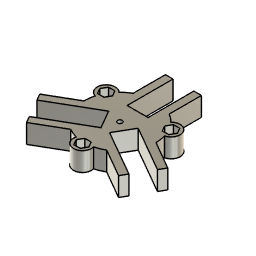
Gripper Assembly v1 (Autodesk Fusion 360 archive; units mm, degrees)
design "Front base"
Autodesk Fusion 360 part; units mm, degrees
sketch "Sketch1" plane through (0, 0, 0) normal (0, 0, 1) x (1, 0, 0)
  line L0 (5, 35) -> (45, 35)
  line L1 (45, 35) -> (45, -135.4224)
  line L2 (5, -135.4224) -> (5, 35)
  spline S0 degree 5 poles (45, -135.4224) (45.4605, -135.6915) (46.3795, -136.2324) (47.752, -137.0519) (49.5701, -138.1606) (51.8226, -139.5739) (54.0546, -141.0154) (56.2658, -142.4857) (58.4561, -143.9858) (60.6259, -145.5165) (62.7755, -147.0783) (64.9051, -148.6715) (67.0143, -150.296) (69.1022, -151.9513) (71.1668, -153.6357) (73.2054, -155.3473) (75.2154, -157.0838) (77.194, -158.8431) (79.1392, -160.6231) (81.0502, -162.4223) (82.9268, -164.2396) (84.4008, -165.7074) (85.491, -166.8158) (86.2111, -167.5582) (86.5694, -167.9302) knots 0 0 0 0 0 0 0.05 0.1 0.15 0.2 0.25 0.3 0.35 0.4 0.45 0.5 0.55 0.6 0.65 0.7 0.75 0.8 0.85 0.9 0.95 1 1 1 1 1 1
  circle A0 centre (121, -201) radius 17.4626
  line L3 (287.62, -385.23) -> (140, -300)
  line L4 (119.9736, -334.6861) -> (267.6136, -419.8616)
  line L5 (267.6136, -419.8616) -> (287.62, -385.23)
  line L6 (119.9736, -334.6861) -> (27.9247, -281.5818)
  line L7 (27.9247, -281.5818) -> (-27.2814, -377.2739)
  line L8 (-27.2814, -377.2739) -> (212.617, -515.1318)
  line L9 (212.617, -515.1318) -> (192.6182, -549.7743)
  line L10 (192.6182, -549.7743) -> (45.092, -464.6088)
  line L11 (5, -135.4224) -> (5, -206.756)
  line L12 (-50, -206.756) -> (5, -206.756)
  spline S1 degree 5 poles (132.5048, -247.3327) (132.6447, -247.7867) (132.9219, -248.702) (133.3302, -250.0971) (133.8594, -252.0018) (134.4952, -254.4571) (135.1045, -256.9868) (135.6863, -259.5888) (136.2394, -262.2585) (136.7623, -264.9875) (137.2534, -267.7647) (137.711, -270.5775) (138.133, -273.4114) (138.5175, -276.2513) (138.8621, -279.082) (139.1649, -281.8886) (139.4238, -284.6572) (139.6373, -287.3762) (139.8044, -290.0362) (139.9248, -292.6319) (139.999, -295.1607) (140.0219, -297.1299) (140.0188, -298.5766) (140.0078, -299.5278) (140, -300) knots 0 0 0 0 0 0 0.05 0.1 0.15 0.2 0.25 0.3 0.35 0.4 0.45 0.5 0.55 0.6 0.65 0.7 0.75 0.8 0.85 0.9 0.95 1 1 1 1 1 1
  spline S2 degree 5 poles (45.092, -464.6088) (44.6241, -464.8703) (43.6871, -465.3905) (42.2779, -466.1627) (40.3917, -467.1758) (38.0214, -468.414) (35.6384, -469.6236) (33.2422, -470.8036) (30.8324, -471.9529) (28.4086, -473.0708) (25.9704, -474.1561) (23.5176, -475.208) (21.0501, -476.2257) (18.568, -477.2083) (16.0719, -478.1551) (13.5623, -479.0659) (11.0402, -479.9402) (8.5062, -480.7781) (5.9613, -481.5796) (3.4059, -482.3453) (0.8406, -483.0761) (-1.2193, -483.6331) (-2.7685, -484.0357) (-3.8032, -484.2974) (-4.321, -484.4265) knots 0 0 0 0 0 0 0.05 0.1 0.15 0.2 0.25 0.3 0.35 0.4 0.45 0.5 0.55 0.6 0.65 0.7 0.75 0.8 0.85 0.9 0.95 1 1 1 1 1 1
  arc A1 (132.5048, -247.3327) -> (86.5694, -167.9302) centre (121, -201) ccw
  arc A2 (-50, -545.0131) -> (-4.321, -484.4265) centre (-50, -497.5) ccw
  arc A3 (-50, -515) -> (-50, -480) centre (-50, -497.5) ccw
  line L13 (-145, 35) -> (-145, -135.4224)
  line L14 (-105, 35) -> (-145, 35)
  line L15 (-105, -135.4224) -> (-105, 35)
  line L16 (-105, -135.4224) -> (-105, -206.756)
  line L17 (-50, -206.756) -> (-105, -206.756)
  line L18 (-219.9736, -334.6861) -> (-367.6136, -419.8616)
  line L19 (-219.9736, -334.6861) -> (-127.9247, -281.5818)
  arc A4 (-186.5694, -167.9302) -> (-232.5048, -247.3327) centre (-221, -201) ccw
  spline S3 degree 5 poles (-145, -135.4224) (-145.4605, -135.6915) (-146.3795, -136.2324) (-147.752, -137.0519) (-149.5701, -138.1606) (-151.8226, -139.5739) (-154.0546, -141.0154) (-156.2658, -142.4857) (-158.4561, -143.9858) (-160.6259, -145.5165) (-162.7755, -147.0783) (-164.9051, -148.6715) (-167.0143, -150.296) (-169.1022, -151.9513) (-171.1668, -153.6357) (-173.2054, -155.3473) (-175.2154, -157.0838) (-177.194, -158.8431) (-179.1392, -160.6231) (-181.0502, -162.4223) (-182.9268, -164.2396) (-184.4008, -165.7074) (-185.491, -166.8158) (-186.2111, -167.5582) (-186.5694, -167.9302) knots 0 0 0 0 0 0 0.05 0.1 0.15 0.2 0.25 0.3 0.35 0.4 0.45 0.5 0.55 0.6 0.65 0.7 0.75 0.8 0.85 0.9 0.95 1 1 1 1 1 1
  line L20 (40.1828, -132.6073) -> (49.8172, -138.2376)
  line L21 (82.7521, -163.9673) -> (90.3868, -171.893)
  line L22 (-140.1828, -132.6073) -> (-149.8172, -138.2376)
  line L23 (-182.7521, -163.9673) -> (-190.3868, -171.893)
  spline S4 degree 5 poles (-232.5048, -247.3327) (-232.6447, -247.7867) (-232.9219, -248.702) (-233.3302, -250.0971) (-233.8594, -252.0018) (-234.4952, -254.4571) (-235.1045, -256.9868) (-235.6863, -259.5888) (-236.2394, -262.2585) (-236.7623, -264.9875) (-237.2534, -267.7647) (-237.711, -270.5775) (-238.133, -273.4114) (-238.5175, -276.2513) (-238.8621, -279.082) (-239.1649, -281.8886) (-239.4238, -284.6572) (-239.6373, -287.3762) (-239.8044, -290.0362) (-239.9248, -292.6319) (-239.999, -295.1607) (-240.0219, -297.1299) (-240.0188, -298.5766) (-240.0078, -299.5278) (-240, -300) knots 0 0 0 0 0 0 0.05 0.1 0.15 0.2 0.25 0.3 0.35 0.4 0.45 0.5 0.55 0.6 0.65 0.7 0.75 0.8 0.85 0.9 0.95 1 1 1 1 1 1
  line L24 (130.9887, -242.4116) -> (134.0209, -252.2537)
  line L25 (140.0843, -294.8664) -> (139.9157, -305.1336)
  line L26 (-230.9887, -242.4116) -> (-234.0209, -252.2537)
  line L27 (-240.0843, -294.8664) -> (-239.9157, -305.1336)
  line L28 (-387.62, -385.23) -> (-240, -300)
  line L29 (-367.6136, -419.8616) -> (-387.62, -385.23)
  line L30 (-127.9247, -281.5818) -> (-72.7186, -377.2739)
  line L31 (-72.7186, -377.2739) -> (-312.617, -515.1318)
  line L32 (-312.617, -515.1318) -> (-292.6182, -549.7743)
  line L33 (-292.6182, -549.7743) -> (-145.092, -464.6088)
  spline S5 degree 5 poles (-145.092, -464.6088) (-144.6241, -464.8703) (-143.6871, -465.3905) (-142.2779, -466.1627) (-140.3917, -467.1758) (-138.0214, -468.414) (-135.6384, -469.6236) (-133.2422, -470.8036) (-130.8324, -471.9529) (-128.4086, -473.0708) (-125.9704, -474.1561) (-123.5176, -475.208) (-121.0501, -476.2257) (-118.568, -477.2083) (-116.0719, -478.1551) (-113.5623, -479.0659) (-111.0402, -479.9402) (-108.5062, -480.7781) (-105.9613, -481.5796) (-103.4059, -482.3453) (-100.8406, -483.0761) (-98.7807, -483.6331) (-97.2315, -484.0357) (-96.1968, -484.2974) (-95.679, -484.4265) knots 0 0 0 0 0 0 0.05 0.1 0.15 0.2 0.25 0.3 0.35 0.4 0.45 0.5 0.55 0.6 0.65 0.7 0.75 0.8 0.85 0.9 0.95 1 1 1 1 1 1
  line L34 (49.9585, -461.8889) -> (40.2255, -467.3286)
  line L35 (1.0783, -483.0799) -> (-9.7202, -485.7731)
  line L36 (-149.9585, -461.8889) -> (-140.2255, -467.3286)
  line L37 (-101.0783, -483.0799) -> (-90.2798, -485.7731)
  arc A5 (-95.679, -484.4265) -> (-50, -545.0131) centre (-50, -497.5) ccw
  arc A6 (-50, -480) -> (-50, -515) centre (-50, -497.5) ccw
  circle A7 centre (-221, -201) radius 17.4626
  circle A8 centre (-50, -300) radius 12.5
  line L38 (137.782, -230.2475) -> (154.5192, -201.2524)
  line L39 (154.5192, -201.2524) -> (137.7773, -172.2599)
  line L40 (137.7773, -172.2599) -> (104.2982, -172.2626)
  line L41 (104.2982, -172.2626) -> (87.561, -201.2578)
  line L42 (87.561, -201.2578) -> (104.3029, -230.2502)
  line L43 (104.3029, -230.2502) -> (137.782, -230.2475)
  line L44 (-204.2982, -172.2626) -> (-187.561, -201.2578)
  line L45 (-187.561, -201.2578) -> (-204.3029, -230.2502)
  line L46 (-204.3029, -230.2502) -> (-237.782, -230.2475)
  line L47 (-237.782, -230.2475) -> (-254.5192, -201.2524)
  line L48 (-254.5192, -201.2524) -> (-237.7773, -172.2599)
  line L49 (-237.7773, -172.2599) -> (-204.2982, -172.2626)
  line L50 (-33.2504, -526.5073) -> (-16.5012, -497.5063)
  line L51 (-16.5012, -497.5063) -> (-33.2422, -468.5005)
  line L52 (-33.2422, -468.5005) -> (-66.7325, -468.4957)
  line L53 (-66.7325, -468.4957) -> (-83.4817, -497.4968)
  line L54 (-83.4817, -497.4968) -> (-66.7407, -526.5025)
  line L55 (-66.7407, -526.5025) -> (-33.2504, -526.5073)
  point P0 (56.3101, -142.5266)
  point P1 (67.0964, -150.3721)
  point P2 (77.3051, -158.9561)
  point P3 (135.5465, -258.9948)
  point P4 (138.1258, -273.4283)
  point P5 (139.6709, -288.0188)
  point P6 (33.22, -470.805)
  point P7 (21.0316, -476.2229)
  point P8 (8.4925, -480.7725)
  point P9 (-156.3101, -142.5266)
  point P10 (-167.0964, -150.3721)
  point P11 (-177.3051, -158.9561)
  point P12 (-235.5465, -258.9948)
  point P13 (-238.1258, -273.4283)
  point P14 (-239.6709, -288.0188)
  point P15 (-133.22, -470.805)
  point P16 (-121.0316, -476.2229)
  point P17 (-108.4925, -480.7725)
  point P18 (121.0401, -201.2551)
  point P19 (-49.9914, -497.5015)
  dimension "d4" = 25
  constraint horizontal L0
  constraint vertical L1
  constraint vertical L2
  constraint concentric A0 A1
  constraint perpendicular L6 L7
  constraint perpendicular L9 L10
  constraint concentric A2 A3
  constraint perpendicular L11 L12
  constraint midpoint L1.end L20
  constraint midpoint S0.end L21
  constraint midpoint S1.start L24
  constraint midpoint L3.end L25
  constraint midpoint L10.end L34
  constraint midpoint S2.end L35
  measures "d4" diameter of A8
extrude "Extrude2" add sketch "Sketch1" along normal blind 100 contours L0 L1 L2 S0 L3 L4 L5 L6 L7 L8 L9 L10 L11 L12 S1 S2 A1 A2 L13 L14 L15 L16 L17 L18 L19 A4 S3 S4 L28 L29 L30 L31 L32 L33 S5 A5
scale "Scale2" factor 0.2 about (86.5694, -167.9302, 100) bodies 1

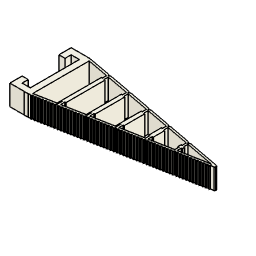
design "CORRUGATED ADAPTIVE FINGER"
Autodesk Fusion 360 part; units mm, degrees
other "Base Mesh Feature1"
sketch "Sketch1" plane through (0, 0, 0) normal (0, 0, 1) x (1, 0, 0)
  line L0 (-20, 150) -> (0, 150)
  line L1 (-0.0012, -150.0012) -> (-19.994, -150.0012)
  line L2 (-90, 150) -> (-20, 150)
  line L3 (-19.994, 120) -> (-60, 120)
  line L4 (-90, 120) -> (-90, 150)
  line L5 (-90, 120) -> (-90, 90)
  line L6 (-90, 90) -> (-60, 90)
  line L7 (-60, 90) -> (-60, 120)
  line L8 (-90, -90) -> (-60, -90)
  line L9 (-60, -90) -> (-60, -120)
  line L10 (-90, -120) -> (-90, -90)
  line L11 (-19.994, -120) -> (-60, -120)
  line L12 (-90, -120) -> (-90, -150)
  line L13 (-90, -150) -> (-19.994, -150)
  line L14 (162.7867, 120.1326) -> (764.7489, 6.3258)
  line L15 (768.431, -1.1614) -> (768.4129, 1.9305)
  line L16 (11.0558, -148.3913) -> (14.7932, -152.3145)
  line L17 (14.7932, -152.3145) -> (16.416, -147.4373)
  line L18 (28.359, -149.753) -> (29.9819, -144.8758)
  line L19 (24.6216, -145.8298) -> (28.359, -149.753)
  line L20 (41.9249, -147.1915) -> (43.5477, -142.3143)
  line L21 (38.1874, -143.2682) -> (41.9249, -147.1915)
  line L22 (55.4907, -144.6299) -> (57.1135, -139.7527)
  line L23 (51.7533, -140.7067) -> (55.4907, -144.6299)
  line L24 (69.0565, -142.0684) -> (70.6794, -137.1912)
  line L25 (65.3191, -138.1452) -> (69.0565, -142.0684)
  line L26 (82.6224, -139.5069) -> (84.2452, -134.6297)
  line L27 (78.885, -135.5837) -> (82.6224, -139.5069)
  line L28 (96.1882, -136.9454) -> (97.811, -132.0682)
  line L29 (92.4508, -133.0221) -> (96.1882, -136.9454)
  line L30 (109.754, -134.3838) -> (111.5052, -129.1209)
  line L31 (106.0166, -130.4606) -> (109.754, -134.3838)
  line L32 (123.3199, -131.8223) -> (124.9427, -126.9451)
  line L33 (119.2419, -127.5416) -> (123.3199, -131.8223)
  line L34 (136.8857, -129.2608) -> (138.5086, -124.3836)
  line L35 (133.1483, -125.3376) -> (136.8857, -129.2608)
  line L36 (150.4516, -126.6993) -> (152.0744, -121.8221)
  line L37 (146.7141, -122.776) -> (150.4516, -126.6993)
  line L38 (164.0174, -124.1377) -> (165.6402, -119.2605)
  line L39 (160.28, -120.2145) -> (164.0174, -124.1377)
  line L40 (177.5832, -121.5762) -> (179.2061, -116.699)
  line L41 (173.8458, -117.653) -> (177.5832, -121.5762)
  line L42 (191.1491, -119.0147) -> (192.7719, -114.1375)
  line L43 (187.4117, -115.0915) -> (191.1491, -119.0147)
  line L44 (204.7149, -116.4532) -> (206.3377, -111.576)
  line L45 (200.9775, -112.5299) -> (204.7149, -116.4532)
  line L46 (218.2807, -113.8916) -> (219.9036, -109.0144)
  line L47 (214.5433, -109.9684) -> (218.2807, -113.8916)
  line L48 (231.8466, -111.3301) -> (233.5929, -106.0817)
  line L49 (228.1092, -107.4069) -> (231.8466, -111.3301)
  line L50 (245.4124, -108.7686) -> (247.0353, -103.8914)
  line L51 (241.4011, -104.5578) -> (245.4124, -108.7686)
  line L52 (258.9783, -106.2071) -> (260.6011, -101.3298)
  line L53 (255.2408, -102.2838) -> (258.9783, -106.2071)
  line L54 (272.5441, -103.6455) -> (274.1669, -98.7683)
  line L55 (268.8067, -99.7223) -> (272.5441, -103.6455)
  line L56 (286.1099, -101.084) -> (287.7328, -96.2068)
  line L57 (282.3725, -97.1608) -> (286.1099, -101.084)
  line L58 (299.6758, -98.5225) -> (301.2986, -93.6453)
  line L59 (295.9384, -94.5993) -> (299.6758, -98.5225)
  line L60 (313.2416, -95.9609) -> (314.8644, -91.0837)
  line L61 (309.5042, -92.0377) -> (313.2416, -95.9609)
  line L62 (326.8074, -93.3994) -> (328.4303, -88.5222)
  line L63 (323.07, -89.4762) -> (326.8074, -93.3994)
  line L64 (340.3733, -90.8379) -> (341.9961, -85.9607)
  line L65 (336.6359, -86.9147) -> (340.3733, -90.8379)
  line L66 (353.9391, -88.2764) -> (355.6866, -83.0245)
  line L67 (350.2017, -84.3531) -> (353.9391, -88.2764)
  line L68 (367.505, -85.7148) -> (369.1278, -80.8376)
  line L69 (363.5002, -81.5109) -> (367.505, -85.7148)
  line L70 (381.0708, -83.1533) -> (382.6936, -78.2761)
  line L71 (377.3334, -79.2301) -> (381.0708, -83.1533)
  line L72 (394.6366, -80.5918) -> (396.2595, -75.7146)
  line L73 (390.8992, -76.6686) -> (394.6366, -80.5918)
  line L74 (408.2025, -78.0303) -> (409.8253, -73.1531)
  line L75 (404.4651, -74.107) -> (408.2025, -78.0303)
  line L76 (421.7683, -75.4687) -> (423.3911, -70.5915)
  line L77 (418.0309, -71.5455) -> (421.7683, -75.4687)
  line L78 (435.3341, -72.9072) -> (436.957, -68.03)
  line L79 (431.5967, -68.984) -> (435.3341, -72.9072)
  line L80 (448.9, -70.3457) -> (450.5228, -65.4685)
  line L81 (445.1626, -66.4225) -> (448.9, -70.3457)
  line L82 (462.4658, -67.7842) -> (464.0887, -62.907)
  line L83 (458.7284, -63.8609) -> (462.4658, -67.7842)
  line L84 (476.0317, -65.2226) -> (477.8401, -59.7876)
  line L85 (472.2942, -61.2994) -> (476.0317, -65.2226)
  line L86 (489.5975, -62.6611) -> (491.2203, -57.7839)
  line L87 (485.4849, -58.3441) -> (489.5975, -62.6611)
  line L88 (503.1633, -60.0996) -> (504.7862, -55.2224)
  line L89 (499.4259, -56.1764) -> (503.1633, -60.0996)
  line L90 (516.7292, -57.5381) -> (518.352, -52.6608)
  line L91 (512.9918, -53.6148) -> (516.7292, -57.5381)
  line L92 (530.295, -54.9765) -> (531.9178, -50.0993)
  line L93 (526.5576, -51.0533) -> (530.295, -54.9765)
  line L94 (543.8608, -52.415) -> (545.4837, -47.5378)
  line L95 (540.1234, -48.4918) -> (543.8608, -52.415)
  line L96 (557.4267, -49.8535) -> (559.0495, -44.9763)
  line L97 (553.6893, -45.9303) -> (557.4267, -49.8535)
  line L98 (570.9925, -47.292) -> (572.6154, -42.4147)
  line L99 (567.2551, -43.3687) -> (570.9925, -47.292)
  line L100 (584.5584, -44.7304) -> (586.1812, -39.8532)
  line L101 (580.8209, -40.8072) -> (584.5584, -44.7304)
  line L102 (598.1242, -42.1689) -> (599.9326, -36.7339)
  line L103 (594.3868, -38.2457) -> (598.1242, -42.1689)
  line L104 (611.69, -39.6074) -> (613.3129, -34.7302)
  line L105 (607.5775, -35.2904) -> (611.69, -39.6074)
  line L106 (625.2559, -37.0458) -> (626.8787, -32.1686)
  line L107 (621.5185, -33.1226) -> (625.2559, -37.0458)
  line L108 (638.8217, -34.4843) -> (640.4445, -29.6071)
  line L109 (635.0843, -30.5611) -> (638.8217, -34.4843)
  line L110 (652.3875, -31.9228) -> (654.0104, -27.0456)
  line L111 (648.6501, -27.9996) -> (652.3875, -31.9228)
  line L112 (665.9534, -29.3613) -> (667.5762, -24.4841)
  line L113 (662.216, -25.438) -> (665.9534, -29.3613)
  line L114 (679.5192, -26.7997) -> (681.1421, -21.9225)
  line L115 (675.7818, -22.8765) -> (679.5192, -26.7997)
  line L116 (693.0851, -24.2382) -> (694.7079, -19.361)
  line L117 (689.3476, -20.315) -> (693.0851, -24.2382)
  line L118 (706.6509, -21.6767) -> (708.2737, -16.7995)
  line L119 (702.9135, -17.7535) -> (706.6509, -21.6767)
  line L120 (720.2167, -19.1152) -> (721.8396, -14.238)
  line L121 (716.4793, -15.1919) -> (720.2167, -19.1152)
  line L122 (733.7826, -16.5536) -> (735.4054, -11.6764)
  line L123 (730.0452, -12.6304) -> (733.7826, -16.5536)
  line L124 (747.3484, -13.9921) -> (749.1569, -8.5571)
  line L125 (743.611, -10.0689) -> (747.3484, -13.9921)
  line L126 (749.1569, -8.5571) -> (764.766, -5.6097)
  line L127 (736.1687, -11.0095) -> (742.7014, -9.776)
  line L128 (722.6029, -13.571) -> (729.1356, -12.3375)
  line L129 (709.037, -16.1326) -> (715.5697, -14.8991)
  line L130 (695.4712, -18.6941) -> (702.0039, -17.4606)
  line L131 (681.9054, -21.2556) -> (688.4381, -20.0221)
  line L132 (668.3395, -23.8171) -> (674.8722, -22.5836)
  line L133 (654.7737, -26.3787) -> (661.3064, -25.1452)
  line L134 (641.2079, -28.9402) -> (647.7405, -27.7067)
  line L135 (627.642, -31.5017) -> (634.1747, -30.2682)
  line L136 (614.0762, -34.0633) -> (620.6089, -32.8297)
  line L137 (586.9445, -39.1863) -> (593.4772, -37.9528)
  line L138 (573.3787, -41.7478) -> (579.9114, -40.5143)
  line L139 (559.8128, -44.3094) -> (566.3455, -43.0758)
  line L140 (546.247, -46.8709) -> (552.7797, -45.6374)
  line L141 (532.6812, -49.4324) -> (539.2138, -48.1989)
  line L142 (519.1153, -51.9939) -> (525.648, -50.7604)
  line L143 (505.5495, -54.5555) -> (512.0822, -53.3219)
  line L144 (491.9836, -57.117) -> (498.5163, -55.8835)
  line L145 (464.852, -62.24) -> (471.3847, -61.0065)
  line L146 (451.2861, -64.8016) -> (457.8188, -63.5681)
  line L147 (437.7203, -67.3631) -> (444.253, -66.1296)
  line L148 (424.1545, -69.9246) -> (430.6871, -68.6911)
  line L149 (410.5886, -72.4861) -> (417.1213, -71.2526)
  line L150 (397.0228, -75.0477) -> (403.5555, -73.8142)
  line L151 (383.4569, -77.6092) -> (389.9896, -76.3757)
  line L152 (9.9848, -148.1289) -> (10.1462, -148.0984)
  line L153 (17.1793, -146.7704) -> (23.712, -145.5369)
  line L154 (30.7452, -144.2089) -> (37.2778, -142.9754)
  line L155 (44.311, -141.6474) -> (50.8437, -140.4138)
  line L156 (57.8768, -139.0858) -> (64.4095, -137.8523)
  line L157 (71.4427, -136.5243) -> (77.9754, -135.2908)
  line L158 (85.0085, -133.9628) -> (91.5412, -132.7293)
  line L159 (98.5744, -131.4012) -> (105.107, -130.1677)
  line L160 (125.706, -126.2782) -> (132.2387, -125.0447)
  line L161 (139.2719, -123.7167) -> (145.8045, -122.4832)
  line L162 (152.8377, -121.1551) -> (159.3704, -119.9216)
  line L163 (166.4035, -118.5936) -> (172.9362, -117.3601)
  line L164 (179.9694, -116.0321) -> (186.5021, -114.7986)
  line L165 (193.5352, -113.4706) -> (200.0679, -112.2371)
  line L166 (207.1011, -110.909) -> (213.6337, -109.6755)
  line L167 (369.8911, -80.1707) -> (376.4238, -78.9372)
  line L168 (342.7594, -85.2938) -> (349.2921, -84.0603)
  line L169 (329.1936, -87.8553) -> (335.7263, -86.6218)
  line L170 (315.6278, -90.4168) -> (322.1604, -89.1833)
  line L171 (302.0619, -92.9784) -> (308.5946, -91.7448)
  line L172 (288.4961, -95.5399) -> (295.0288, -94.3064)
  line L173 (274.9302, -98.1014) -> (281.4629, -96.8679)
  line L174 (261.3644, -100.6629) -> (267.8971, -99.4294)
  line L175 (247.7986, -103.2245) -> (254.3313, -101.9909)
  line L176 (220.6669, -108.3475) -> (227.1996, -107.114)
  line L177 (-19.994, -150.0012) -> (-19.994, -150)
  line L178 (-19.994, -120) -> (-19.994, 120)
  line L179 (9.9848, -148.1289) -> (-0.0012, -150.0012)
  line L180 (162.7867, 120.1326) -> (0, 150)
  line L181 (10, -137.9994) -> (745.7473, -0.0019)
  line L182 (745.7473, -0.0019) -> (10.003, 137.9556)
  line L183 (10.003, 137.9556) -> (10, -137.9994)
  line L184 (607.5775, -35.2904) -> (602, -32)
  line L185 (602, -32) -> (599.9326, -36.7339)
  line L186 (485.4849, -58.3441) -> (480.1362, -55.5815)
  line L187 (480.1362, -55.5815) -> (477.8401, -59.7876)
  line L188 (363.2553, -81.323) -> (359, -79)
  line L189 (359, -79) -> (355.8723, -82.694)
  line L190 (241.1723, -104.3789) -> (237, -102)
  line L191 (237, -102) -> (233.7832, -105.7459)
  line L192 (119.1693, -127.4727) -> (115.3849, -124.2227)
  line L193 (115.3849, -124.2227) -> (111.6766, -128.8078)
  arc A0 (743.611, -10.0689) -> (742.7014, -9.776) centre (742.8869, -10.7586) ccw
  arc A1 (736.1687, -11.0095) -> (735.4054, -11.6764) centre (736.3543, -11.9922) ccw
  arc A2 (730.0452, -12.6304) -> (729.1356, -12.3375) centre (729.3211, -13.3202) ccw
  arc A3 (722.6029, -13.571) -> (721.8396, -14.238) centre (722.7884, -14.5537) ccw
  arc A4 (716.4793, -15.1919) -> (715.5697, -14.8991) centre (715.7553, -15.8817) ccw
  arc A5 (709.037, -16.1326) -> (708.2737, -16.7995) centre (709.2226, -17.1152) ccw
  arc A6 (702.9135, -17.7535) -> (702.0039, -17.4606) centre (702.1894, -18.4432) ccw
  arc A7 (695.4712, -18.6941) -> (694.7079, -19.361) centre (695.6567, -19.6767) ccw
  arc A8 (689.3476, -20.315) -> (688.4381, -20.0221) centre (688.6236, -21.0047) ccw
  arc A9 (681.9054, -21.2556) -> (681.1421, -21.9225) centre (682.0909, -22.2383) ccw
  arc A10 (675.7818, -22.8765) -> (674.8722, -22.5836) centre (675.0578, -23.5663) ccw
  arc A11 (668.3395, -23.8171) -> (667.5762, -24.4841) centre (668.5251, -24.7998) ccw
  arc A12 (662.216, -25.438) -> (661.3064, -25.1452) centre (661.4919, -26.1278) ccw
  arc A13 (654.7737, -26.3787) -> (654.0104, -27.0456) centre (654.9592, -27.3613) ccw
  arc A14 (648.6501, -27.9996) -> (647.7405, -27.7067) centre (647.9261, -28.6893) ccw
  arc A15 (641.2079, -28.9402) -> (640.4445, -29.6071) centre (641.3934, -29.9228) ccw
  arc A16 (635.0843, -30.5611) -> (634.1747, -30.2682) centre (634.3602, -31.2508) ccw
  arc A17 (627.642, -31.5017) -> (626.8787, -32.1686) centre (627.8276, -32.4844) ccw
  arc A18 (621.5185, -33.1226) -> (620.6089, -32.8297) centre (620.7944, -33.8124) ccw
  arc A19 (614.0762, -34.0633) -> (613.3129, -34.7302) centre (614.2617, -35.0459) ccw
  arc A20 (594.3868, -38.2457) -> (593.4772, -37.9528) centre (593.6627, -38.9354) ccw
  arc A21 (586.9445, -39.1863) -> (586.1812, -39.8532) centre (587.13, -40.1689) ccw
  arc A22 (580.8209, -40.8072) -> (579.9114, -40.5143) centre (580.0969, -41.497) ccw
  arc A23 (573.3787, -41.7478) -> (572.6154, -42.4147) centre (573.5642, -42.7305) ccw
  arc A24 (567.2551, -43.3687) -> (566.3455, -43.0758) centre (566.5311, -44.0585) ccw
  arc A25 (559.8128, -44.3094) -> (559.0495, -44.9763) centre (559.9984, -45.292) ccw
  arc A26 (553.6893, -45.9303) -> (552.7797, -45.6374) centre (552.9652, -46.62) ccw
  arc A27 (546.247, -46.8709) -> (545.4837, -47.5378) centre (546.4325, -47.8535) ccw
  arc A28 (540.1234, -48.4918) -> (539.2138, -48.1989) centre (539.3994, -49.1815) ccw
  arc A29 (532.6812, -49.4324) -> (531.9178, -50.0993) centre (532.8667, -50.415) ccw
  arc A30 (526.5576, -51.0533) -> (525.648, -50.7604) centre (525.8335, -51.7431) ccw
  arc A31 (519.1153, -51.9939) -> (518.352, -52.6608) centre (519.3009, -52.9766) ccw
  arc A32 (512.9918, -53.6148) -> (512.0822, -53.3219) centre (512.2677, -54.3046) ccw
  arc A33 (505.5495, -54.5555) -> (504.7862, -55.2224) centre (505.735, -55.5381) ccw
  arc A34 (499.4259, -56.1764) -> (498.5163, -55.8835) centre (498.7019, -56.8661) ccw
  arc A35 (491.9836, -57.117) -> (491.2203, -57.7839) centre (492.1692, -58.0996) ccw
  arc A36 (472.2942, -61.2994) -> (471.3847, -61.0065) centre (471.5702, -61.9892) ccw
  arc A37 (464.852, -62.24) -> (464.0887, -62.907) centre (465.0375, -63.2227) ccw
  arc A38 (458.7284, -63.8609) -> (457.8188, -63.5681) centre (458.0044, -64.5507) ccw
  arc A39 (451.2861, -64.8016) -> (450.5228, -65.4685) centre (451.4717, -65.7842) ccw
  arc A40 (445.1626, -66.4225) -> (444.253, -66.1296) centre (444.4385, -67.1122) ccw
  arc A41 (437.7203, -67.3631) -> (436.957, -68.03) centre (437.9058, -68.3457) ccw
  arc A42 (431.5967, -68.984) -> (430.6871, -68.6911) centre (430.8727, -69.6737) ccw
  arc A43 (424.1545, -69.9246) -> (423.3911, -70.5915) centre (424.34, -70.9073) ccw
  arc A44 (418.0309, -71.5455) -> (417.1213, -71.2526) centre (417.3068, -72.2353) ccw
  arc A45 (410.5886, -72.4861) -> (409.8253, -73.1531) centre (410.7742, -73.4688) ccw
  arc A46 (404.4651, -74.107) -> (403.5555, -73.8142) centre (403.741, -74.7968) ccw
  arc A47 (397.0228, -75.0477) -> (396.2595, -75.7146) centre (397.2083, -76.0303) ccw
  arc A48 (390.8992, -76.6686) -> (389.9896, -76.3757) centre (390.1752, -77.3583) ccw
  arc A49 (383.4569, -77.6092) -> (382.6936, -78.2761) centre (383.6425, -78.5918) ccw
  arc A50 (377.3334, -79.2301) -> (376.4238, -78.9372) centre (376.6093, -79.9198) ccw
  arc A51 (369.8911, -80.1707) -> (369.1278, -80.8376) centre (370.0766, -81.1534) ccw
  arc A52 (350.2017, -84.3531) -> (349.2921, -84.0603) centre (349.4777, -85.0429) ccw
  arc A53 (342.7594, -85.2938) -> (341.9961, -85.9607) centre (342.945, -86.2764) ccw
  arc A54 (336.6359, -86.9147) -> (335.7263, -86.6218) centre (335.9118, -87.6044) ccw
  arc A55 (363.5002, -81.5109) -> (363.2553, -81.323) centre (362.7761, -82.2007) ccw
  arc A56 (355.8723, -82.694) -> (355.6866, -83.0245) centre (356.6355, -83.3402) ccw
  arc A57 (329.1936, -87.8553) -> (328.4303, -88.5222) centre (329.3791, -88.8379) ccw
  arc A58 (323.07, -89.4762) -> (322.1604, -89.1833) centre (322.346, -90.166) ccw
  arc A59 (315.6278, -90.4168) -> (314.8644, -91.0837) centre (315.8133, -91.3995) ccw
  arc A60 (309.5042, -92.0377) -> (308.5946, -91.7448) centre (308.7801, -92.7275) ccw
  arc A61 (302.0619, -92.9784) -> (301.2986, -93.6453) centre (302.2475, -93.961) ccw
  arc A62 (295.9384, -94.5993) -> (295.0288, -94.3064) centre (295.2143, -95.289) ccw
  arc A63 (288.4961, -95.5399) -> (287.7328, -96.2068) centre (288.6816, -96.5225) ccw
  arc A64 (282.3725, -97.1608) -> (281.4629, -96.8679) centre (281.6485, -97.8505) ccw
  arc A65 (274.9302, -98.1014) -> (274.1669, -98.7683) centre (275.1158, -99.084) ccw
  arc A66 (268.8067, -99.7223) -> (267.8971, -99.4294) centre (268.0826, -100.4121) ccw
  arc A67 (261.3644, -100.6629) -> (260.6011, -101.3298) centre (261.5499, -101.6456) ccw
  arc A68 (255.2408, -102.2838) -> (254.3313, -101.9909) centre (254.5168, -102.9736) ccw
  arc A69 (247.7986, -103.2245) -> (247.0353, -103.8914) centre (247.9841, -104.2071) ccw
  arc A70 (241.4011, -104.5578) -> (241.1723, -104.3789) centre (240.677, -105.2476) ccw
  arc A71 (233.7832, -105.7459) -> (233.5929, -106.0817) centre (234.5418, -106.3974) ccw
  arc A72 (228.1092, -107.4069) -> (227.1996, -107.114) centre (227.3851, -108.0966) ccw
  arc A73 (220.6669, -108.3475) -> (219.9036, -109.0144) centre (220.8524, -109.3301) ccw
  arc A74 (214.5433, -109.9684) -> (213.6337, -109.6755) centre (213.8193, -110.6582) ccw
  arc A75 (207.1011, -110.909) -> (206.3377, -111.576) centre (207.2866, -111.8917) ccw
  arc A76 (200.9775, -112.5299) -> (200.0679, -112.2371) centre (200.2534, -113.2197) ccw
  arc A77 (193.5352, -113.4706) -> (192.7719, -114.1375) centre (193.7208, -114.4532) ccw
  arc A78 (187.4117, -115.0915) -> (186.5021, -114.7986) centre (186.6876, -115.7812) ccw
  arc A79 (179.9694, -116.0321) -> (179.2061, -116.699) centre (180.1549, -117.0147) ccw
  arc A80 (173.8458, -117.653) -> (172.9362, -117.3601) centre (173.1218, -118.3427) ccw
  arc A81 (166.4035, -118.5936) -> (165.6402, -119.2605) centre (166.5891, -119.5763) ccw
  arc A82 (160.28, -120.2145) -> (159.3704, -119.9216) centre (159.5559, -120.9043) ccw
  arc A83 (152.8377, -121.1551) -> (152.0744, -121.8221) centre (153.0232, -122.1378) ccw
  arc A84 (146.7141, -122.776) -> (145.8045, -122.4832) centre (145.9901, -123.4658) ccw
  arc A85 (139.2719, -123.7167) -> (138.5086, -124.3836) centre (139.4574, -124.6993) ccw
  arc A86 (133.1483, -125.3376) -> (132.2387, -125.0447) centre (132.4243, -126.0273) ccw
  arc A87 (125.706, -126.2782) -> (124.9427, -126.9451) centre (125.8916, -127.2608) ccw
  arc A88 (119.2419, -127.5416) -> (119.1693, -127.4727) centre (118.5178, -128.2313) ccw
  arc A89 (111.6766, -128.8078) -> (111.5052, -129.1209) centre (112.4541, -129.4366) ccw
  arc A90 (106.0166, -130.4606) -> (105.107, -130.1677) centre (105.2926, -131.1504) ccw
  arc A91 (98.5744, -131.4012) -> (97.811, -132.0682) centre (98.7599, -132.3839) ccw
  arc A92 (92.4508, -133.0221) -> (91.5412, -132.7293) centre (91.7267, -133.7119) ccw
  arc A93 (85.0085, -133.9628) -> (84.2452, -134.6297) centre (85.1941, -134.9454) ccw
  arc A94 (78.885, -135.5837) -> (77.9754, -135.2908) centre (78.1609, -136.2734) ccw
  arc A95 (71.4427, -136.5243) -> (70.6794, -137.1912) centre (71.6282, -137.5069) ccw
  arc A96 (65.3191, -138.1452) -> (64.4095, -137.8523) centre (64.5951, -138.8349) ccw
  arc A97 (57.8768, -139.0858) -> (57.1135, -139.7527) centre (58.0624, -140.0685) ccw
  arc A98 (51.7533, -140.7067) -> (50.8437, -140.4138) centre (51.0292, -141.3965) ccw
  arc A99 (44.311, -141.6474) -> (43.5477, -142.3143) centre (44.4965, -142.63) ccw
  arc A100 (38.1874, -143.2682) -> (37.2778, -142.9754) centre (37.4634, -143.958) ccw
  arc A101 (30.7452, -144.2089) -> (29.9819, -144.8758) centre (30.9307, -145.1915) ccw
  arc A102 (24.6216, -145.8298) -> (23.712, -145.5369) centre (23.8976, -146.5195) ccw
  arc A103 (17.1793, -146.7704) -> (16.416, -147.4373) centre (17.3649, -147.753) ccw
  arc A104 (11.0558, -148.3913) -> (10.1462, -148.0984) centre (10.3317, -149.0811) ccw
  arc A105 (768.4129, 1.9305) -> (764.7489, 6.3258) centre (763.9129, 1.9041) ccw
  arc A106 (764.766, -5.6097) -> (768.431, -1.1614) centre (763.9311, -1.1879) ccw
  line L194 (594.9958, -7.9003) -> (589.99, -8.8391)
  line L195 (589.99, -8.8391) -> (589.99, 8.8532)
  line L196 (589.99, 8.8532) -> (594.9958, 7.917)
  line L197 (605, -6.0399) -> (610.0002, -5.1023)
  line L198 (610.0002, -5.1023) -> (610.0002, 5.1)
  line L199 (610.0002, 5.1) -> (605, 6)
  line L200 (474.9967, -30.4201) -> (469.9586, -31.3651)
  line L201 (469.9586, -31.3651) -> (469.9586, 31.3975)
  line L202 (469.9586, 31.3975) -> (474.9967, 30.4853)
  line L203 (484.9989, 28.5419) -> (490, 27.6)
  line L204 (490, 27.6) -> (490, -27.6)
  line L205 (490, -27.6) -> (484.9989, -28.5172)
  line L206 (354.9916, -52.9111) -> (349.9496, -53.8358)
  line L207 (349.9496, -53.8358) -> (349.9496, 53.9582)
  line L208 (349.9496, 53.9582) -> (354.9916, 52.9552)
  line L209 (365.0033, -51.1307) -> (370.0851, -50.1711)
  line L210 (370.0851, -50.1711) -> (370.0851, 50)
  line L211 (370.0851, 50) -> (365.0033, 51.0109)
  line L212 (234.9803, -75.3997) -> (230, -76.35)
  line L213 (230, 76.35) -> (234.9803, 75.4147)
  line L214 (245.0024, 73.5325) -> (250, 72.6)
  line L215 (250, 72.6) -> (250, -72.6)
  line L216 (250, -72.6) -> (245.0024, -73.5488)
  line L217 (124.9971, 96.0244) -> (124.9995, 116.3929)
  line L218 (114.9893, 97.915) -> (110.0006, 98.8537)
  line L219 (110.0006, 98.8537) -> (109.9772, -98.8618)
  line L220 (109.9772, -98.8618) -> (114.9661, -97.9219)
  line L221 (124.9858, -96.0536) -> (130, -95.1)
  line L222 (130, -95.1) -> (130.0225, 95.0835)
  line L223 (130.0225, 95.0835) -> (124.9971, 96.0244)
  line L224 (605, 26.3892) -> (605, 6)
  line L225 (605, -6.0399) -> (605, -26.4006)
  line L226 (594.9958, -28.277) -> (594.9958, -7.9003)
  line L227 (594.9958, 7.917) -> (594.9958, 28.2651)
  line L228 (484.9989, -48.9082) -> (484.9989, -28.5172)
  line L229 (484.9989, 28.5419) -> (484.9989, 48.8903)
  line L230 (474.9967, -50.7842) -> (474.9967, -30.4201)
  line L231 (474.9967, 30.4853) -> (474.9967, 50.7658)
  line L232 (365.0033, -71.4147) -> (365.0033, -51.1307)
  line L233 (365.0033, 51.0109) -> (365.0033, 71.3904)
  line L234 (354.9916, -73.2925) -> (354.9916, -52.9111)
  line L235 (354.9916, 52.9552) -> (354.9916, 73.2677)
  line L236 (245.0024, -93.9222) -> (245.0024, -73.5488)
  line L237 (245.0024, 73.5325) -> (245.0024, 93.8914)
  line L238 (234.9803, -95.8019) -> (234.9803, -75.3997)
  line L239 (234.9803, 75.4147) -> (234.9803, 95.7707)
  line L240 (230, -76.35) -> (230, 76.35)
  line L241 (114.9637, -118.3123) -> (114.9661, -97.9219)
  line L242 (114.9893, 97.915) -> (114.9917, 118.2694)
  line L243 (124.9858, -96.0536) -> (124.9858, -116.4326)
  line L244 (113.629, 129.1518) -> (119.7911, 123.1363)
  line L245 (119.7911, 123.1363) -> (127.0564, 126.6883)
  line L246 (235.6765, 106.3521) -> (240.0931, 99.757)
  line L247 (240.0931, 99.757) -> (248.5894, 103.9108)
  line L248 (355.824, 83.637) -> (360.6108, 76.4891)
  line L249 (360.6108, 76.4891) -> (369.6575, 81.0217)
  line L250 (475.3542, 61.0387) -> (479.5132, 54.8283)
  line L251 (479.5132, 54.8283) -> (487.3733, 58.7663)
  line L252 (594.9107, 38.4353) -> (599.9126, 30.9663)
  line L253 (599.9126, 30.9663) -> (609.3658, 35.7025)
  dimension "d5" = 1
  dimension "d6" = 4.5
  dimension "d7" = 4.5
  constraint horizontal L0
  constraint horizontal L1
  constraint vertical L177
  constraint horizontal L2
  constraint horizontal L3
  constraint vertical L4
  constraint coincident L3.start L177
  constraint vertical L5
  constraint horizontal L6
  constraint vertical L7
  constraint horizontal L8
  constraint vertical L9
  constraint vertical L10
  constraint horizontal L11
  constraint vertical L12
  constraint horizontal L13
  constraint coincident L11.start L177
  constraint collinear L126 L152
  constraint collinear L127 L152
  constraint collinear L128 L152
  constraint collinear L129 L152
  constraint collinear L130 L152
  constraint collinear L131 L152
  constraint collinear L132 L152
  constraint collinear L133 L152
  constraint collinear L134 L152
  constraint collinear L135 L152
  constraint collinear L136 L152
  constraint collinear L137 L152
  constraint collinear L138 L152
  constraint collinear L139 L152
  constraint collinear L140 L152
  constraint collinear L141 L152
  constraint collinear L142 L152
  constraint collinear L143 L152
  constraint collinear L144 L152
  constraint collinear L145 L152
  constraint collinear L146 L152
  constraint collinear L147 L152
  constraint collinear L148 L152
  constraint collinear L149 L152
  constraint collinear L150 L152
  constraint collinear L151 L152
  constraint collinear L152 L154
  constraint collinear L152 L153
  constraint collinear L154 L155
  constraint collinear L155 L156
  constraint collinear L156 L157
  constraint collinear L157 L158
  constraint collinear L158 L159
  constraint collinear L160 L161
  constraint collinear L161 L162
  constraint collinear L162 L163
  constraint collinear L163 L164
  constraint collinear L164 L165
  constraint collinear L165 L166
  constraint collinear L166 L176
  constraint collinear L167 L176
  constraint collinear L168 L176
  constraint collinear L169 L176
  constraint collinear L170 L176
  constraint collinear L171 L176
  constraint collinear L172 L176
  constraint collinear L173 L176
  constraint collinear L174 L176
  constraint collinear L175 L176
  constraint collinear L177 L178
  constraint perpendicular L187 L188
  constraint perpendicular L191 L192
  constraint tangent L125 A0
  constraint tangent L127 A0
  constraint tangent L122 A1
  constraint tangent L127 A1
  constraint equal A0 A1
  constraint tangent L123 A2
  constraint tangent L128 A2
  constraint equal A0 A2
  constraint tangent L120 A3
  constraint tangent L128 A3
  constraint equal A0 A3
  constraint tangent L121 A4
  constraint tangent L129 A4
  constraint equal A0 A4
  constraint tangent L118 A5
  constraint tangent L129 A5
  constraint equal A0 A5
  constraint tangent L119 A6
  constraint tangent L130 A6
  constraint equal A0 A6
  constraint tangent L116 A7
  constraint tangent L130 A7
  constraint equal A0 A7
  constraint tangent L117 A8
  constraint tangent L131 A8
  constraint equal A0 A8
  constraint tangent L114 A9
  constraint tangent L131 A9
  constraint equal A0 A9
  constraint tangent L115 A10
  constraint tangent L132 A10
  constraint equal A0 A10
  constraint tangent L112 A11
  constraint tangent L132 A11
  constraint equal A0 A11
  constraint tangent L113 A12
  constraint tangent L133 A12
  constraint equal A0 A12
  constraint tangent L110 A13
  constraint tangent L133 A13
  constraint equal A0 A13
  constraint tangent L111 A14
  constraint tangent L134 A14
  constraint equal A0 A14
  constraint tangent L108 A15
  constraint tangent L134 A15
  constraint equal A0 A15
  constraint tangent L109 A16
  constraint tangent L135 A16
  constraint equal A0 A16
  constraint tangent L106 A17
  constraint tangent L135 A17
  constraint equal A0 A17
  constraint tangent L107 A18
  constraint tangent L136 A18
  constraint equal A0 A18
  constraint tangent L104 A19
  constraint tangent L136 A19
  constraint equal A0 A19
  constraint tangent L103 A20
  constraint tangent L137 A20
  constraint equal A0 A20
  constraint tangent L100 A21
  constraint tangent L137 A21
  constraint equal A0 A21
  constraint tangent L101 A22
  constraint tangent L138 A22
  constraint equal A0 A22
  constraint tangent L98 A23
  constraint tangent L138 A23
  constraint equal A0 A23
  constraint tangent L99 A24
  constraint tangent L139 A24
  constraint equal A0 A24
  constraint tangent L96 A25
  constraint tangent L139 A25
  constraint equal A0 A25
  constraint tangent L97 A26
  constraint tangent L140 A26
  constraint equal A0 A26
  constraint tangent L94 A27
  constraint tangent L140 A27
  constraint equal A0 A27
  constraint tangent L95 A28
  constraint tangent L141 A28
  constraint equal A0 A28
  constraint tangent L92 A29
  constraint tangent L141 A29
  constraint equal A0 A29
  constraint tangent L93 A30
  constraint tangent L142 A30
  constraint equal A0 A30
  constraint tangent L90 A31
  constraint tangent L142 A31
  constraint equal A0 A31
  constraint tangent L91 A32
  constraint tangent L143 A32
  constraint equal A0 A32
  constraint tangent L88 A33
  constraint tangent L143 A33
  constraint equal A0 A33
  constraint tangent L89 A34
  constraint tangent L144 A34
  constraint equal A0 A34
  constraint tangent L86 A35
  constraint tangent L144 A35
  constraint equal A0 A35
  constraint tangent L85 A36
  constraint tangent L145 A36
  constraint equal A0 A36
  constraint tangent L82 A37
  constraint tangent L145 A37
  constraint equal A0 A37
  constraint tangent L83 A38
  constraint tangent L146 A38
  constraint equal A0 A38
  constraint tangent L80 A39
  constraint tangent L146 A39
  constraint equal A0 A39
  constraint tangent L81 A40
  constraint tangent L147 A40
  constraint equal A0 A40
  constraint tangent L78 A41
  constraint tangent L147 A41
  constraint equal A0 A41
  constraint tangent L79 A42
  constraint tangent L148 A42
  constraint equal A0 A42
  constraint tangent L76 A43
  constraint tangent L148 A43
  constraint equal A0 A43
  constraint tangent L77 A44
  constraint tangent L149 A44
  constraint equal A0 A44
  constraint tangent L74 A45
  constraint tangent L149 A45
  constraint equal A0 A45
  constraint tangent L75 A46
  constraint tangent L150 A46
  constraint equal A0 A46
  constraint tangent L72 A47
  constraint tangent L150 A47
  constraint equal A0 A47
  constraint tangent L73 A48
  constraint tangent L151 A48
  constraint equal A0 A48
  constraint tangent L70 A49
  constraint tangent L151 A49
  constraint equal A0 A49
  constraint tangent L71 A50
  constraint tangent L167 A50
  constraint equal A0 A50
  constraint tangent L68 A51
  constraint tangent L167 A51
  constraint equal A0 A51
  constraint tangent L67 A52
  constraint tangent L168 A52
  constraint equal A0 A52
  constraint tangent L64 A53
  constraint tangent L168 A53
  constraint equal A0 A53
  constraint tangent L65 A54
  constraint tangent L169 A54
  constraint equal A0 A54
  constraint tangent L69 A55
  constraint tangent L188 A55
  constraint equal A0 A55
  constraint tangent L66 A56
  constraint tangent L189 A56
  constraint equal A0 A56
  constraint tangent L62 A57
  constraint tangent L169 A57
  constraint equal A0 A57
  constraint tangent L63 A58
  constraint tangent L170 A58
  constraint equal A0 A58
  constraint tangent L60 A59
  constraint tangent L170 A59
  constraint equal A0 A59
  constraint tangent L61 A60
  constraint tangent L171 A60
  constraint equal A0 A60
  constraint tangent L58 A61
  constraint tangent L171 A61
  constraint equal A0 A61
  constraint tangent L59 A62
  constraint tangent L172 A62
  constraint equal A0 A62
  constraint tangent L56 A63
  constraint tangent L172 A63
  constraint equal A0 A63
  constraint tangent L57 A64
  constraint tangent L173 A64
  constraint equal A0 A64
  constraint tangent L54 A65
  constraint tangent L173 A65
  constraint equal A0 A65
  constraint tangent L55 A66
  constraint tangent L174 A66
  constraint equal A0 A66
  constraint tangent L52 A67
  constraint tangent L174 A67
  constraint equal A0 A67
  constraint tangent L53 A68
  constraint tangent L175 A68
  constraint equal A0 A68
  constraint tangent L50 A69
  constraint tangent L175 A69
  constraint equal A0 A69
  constraint tangent L51 A70
  constraint tangent L190 A70
  constraint equal A0 A70
  constraint tangent L48 A71
  constraint tangent L191 A71
  constraint equal A0 A71
  constraint tangent L49 A72
  constraint tangent L176 A72
  constraint equal A0 A72
  constraint tangent L46 A73
  constraint tangent L176 A73
  constraint equal A0 A73
  constraint tangent L47 A74
  constraint tangent L166 A74
  constraint equal A0 A74
  constraint tangent L44 A75
  constraint tangent L166 A75
  constraint equal A0 A75
  constraint tangent L45 A76
  constraint tangent L165 A76
  constraint equal A0 A76
  constraint tangent L42 A77
  constraint tangent L165 A77
  constraint equal A0 A77
  constraint tangent L43 A78
  constraint tangent L164 A78
  constraint equal A0 A78
  constraint tangent L40 A79
  constraint tangent L164 A79
  constraint equal A0 A79
  constraint tangent L41 A80
  constraint tangent L163 A80
  constraint equal A0 A80
  constraint tangent L38 A81
  constraint tangent L163 A81
  constraint equal A0 A81
  constraint tangent L39 A82
  constraint tangent L162 A82
  constraint equal A0 A82
  constraint tangent L36 A83
  constraint tangent L162 A83
  constraint equal A0 A83
  constraint tangent L37 A84
  constraint tangent L161 A84
  constraint equal A0 A84
  constraint tangent L34 A85
  constraint tangent L161 A85
  constraint equal A0 A85
  constraint tangent L35 A86
  constraint tangent L160 A86
  constraint equal A0 A86
  constraint tangent L32 A87
  constraint tangent L160 A87
  constraint equal A0 A87
  constraint tangent L33 A88
  constraint tangent L192 A88
  constraint equal A0 A88
  constraint tangent L30 A89
  constraint tangent L193 A89
  constraint equal A0 A89
  constraint tangent L31 A90
  constraint tangent L159 A90
  constraint equal A0 A90
  constraint tangent L28 A91
  constraint tangent L159 A91
  constraint equal A0 A91
  constraint tangent L29 A92
  constraint tangent L158 A92
  constraint equal A0 A92
  constraint tangent L26 A93
  constraint tangent L158 A93
  constraint equal A0 A93
  constraint tangent L27 A94
  constraint tangent L157 A94
  constraint equal A0 A94
  constraint tangent L24 A95
  constraint tangent L157 A95
  constraint equal A0 A95
  constraint tangent L25 A96
  constraint tangent L156 A96
  constraint equal A0 A96
  constraint tangent L22 A97
  constraint tangent L156 A97
  constraint equal A0 A97
  constraint tangent L23 A98
  constraint tangent L155 A98
  constraint equal A0 A98
  constraint tangent L20 A99
  constraint tangent L155 A99
  constraint equal A0 A99
  constraint tangent L21 A100
  constraint tangent L154 A100
  constraint equal A0 A100
  constraint tangent L18 A101
  constraint tangent L154 A101
  constraint equal A0 A101
  constraint tangent L19 A102
  constraint tangent L153 A102
  constraint equal A0 A102
  constraint tangent L17 A103
  constraint tangent L153 A103
  constraint equal A0 A103
  constraint tangent L16 A104
  constraint tangent L152 A104
  constraint equal A0 A104
  constraint tangent L14 A105
  constraint tangent L15 A105
  constraint tangent L126 A106
  constraint tangent L15 A106
  constraint vertical L224
  constraint coincident L181 L225.end
  constraint coincident L182 L224.start
  constraint coincident L181 L226.start
  constraint coincident L182 L227.end
  constraint vertical L226
  constraint parallel L181 L194
  constraint parallel L195 L226
  constraint coincident L196.end L226
  constraint coincident L197.start L224
  constraint parallel L198 L224
  constraint coincident L181 L228.start
  constraint coincident L182 L229.end
  constraint parallel L198 L228
  constraint coincident L181 L230.start
  constraint coincident L182 L231.end
  constraint parallel L228 L230
  constraint parallel L181 L200
  constraint parallel L201 L230
  constraint coincident L202.end L230
  constraint coincident L203.start L228
  constraint parallel L204 L228
  constraint coincident L181 L232.start
  constraint coincident L182 L233.end
  constraint parallel L201 L232
  constraint coincident L181 L234.start
  constraint coincident L182 L235.end
  constraint parallel L232 L234
  constraint parallel L205 L206
  constraint parallel L207 L234
  constraint coincident L208.end L234
  constraint parallel L169 L209
  constraint parallel L210 L232
  constraint coincident L211.end L232
  constraint parallel L208 L211
  constraint coincident L181 L236.start
  constraint coincident L182 L237.end
  constraint parallel L210 L236
  constraint coincident L181 L238.start
  constraint coincident L182 L239.end
  constraint parallel L236 L238
  constraint coincident L213.end L238
  constraint coincident L214.start L236
  constraint parallel L215 L236
  constraint coincident L182 L217.end
  constraint coincident L181 L241.start
  constraint coincident L182 L242.end
  constraint parallel L217 L241
  constraint coincident L218.start L241
  constraint parallel L219 L241
  constraint parallel L217 L222
  constraint collinear L224 L225
  constraint collinear L226 L227
  constraint collinear L228 L229
  constraint collinear L230 L231
  constraint collinear L232 L233
  constraint collinear L234 L235
  constraint collinear L236 L237
  constraint collinear L238 L239
  constraint parallel L215 L240
  constraint collinear L241 L242
  constraint coincident L181 L243.end
  constraint vertical L243
  constraint coincident L180 L244.start
  constraint coincident L180 L245.end
  constraint coincident L14 L246.start
  constraint coincident L14 L247.end
  constraint parallel L245 L247
  constraint coincident L14 L248.start
  constraint parallel L246 L248
  constraint coincident L14 L249.end
  constraint coincident L14 L250.start
  constraint parallel L248 L250
  constraint coincident L14 L251.end
  constraint parallel L249 L251
  constraint coincident L14 L252.start
  constraint parallel L250 L252
  constraint coincident L14 L253.end
  constraint parallel L249 L253
  measures "d5" radius of A0
  measures "d6" radius of A105
  measures "d7" radius of A106
extrude "Extrude1" add sketch "Sketch1" along normal blind 100 contours L0 L1 L2 L3 L4 L5 L6 L7 L8 L9 L10 L11 L12 L13 L14 L15 L16 L17 L18 L19 L20 L21 L22 L23 L24 L25 L26 L27 L28 L29 L30 L31 L32 L33 L34 L35 L36 L37 L38 L39 L40 L41 L42 L43 L44 L45 L46 L47 L48 L49 L50 L51 L52 L53 L54 L55 L56 L57 L58 L59 L60 L61 L62 L63 L64 L65 L66 L67 L68 L69 L70 L71 L72 L73 L74 L75 L76 L77 L78 L79 L80 L81 L82 L83 L84 L85 L86 L87 L88 L89 L90 L91 L92 L93 L94 L95 L96 L97 L98 L99 L100 L101 L102 L103 L104 L105 L106 L107 L108 L109 L110 L111 L112 L113 L114 L115 L116 L117 L118 L119 L120 L121 L122 L123 L124 L125 L126 L127 L128 L129 L130 L131 L132 L133 L134 L135 L136 L137 L138 L139 L140 L141 L142 L143 L144 L145 L146 L147 L148 L149 L150 L151 L152 L153 L154 L155 L156 L157 L158 L159 L160 L161 L162 L163 L164 L165 L166 L167 L168 L169 L170 L171 L172 L173 L174 L175 L176 L178 L179 L180 L184 L185 L186 L187 L188 L189 L190 L191 L192 L193 A0 A1 A2 A3 A4 A5 A6 A7 A8 A9 A10 A11 A12 A13 A14 A15 A16 A17 A18 A19 A20 A21 A22 A23 A24 A25 A26 A27 A28 A29 A30 A31 A32 A33 A34 A35 A36 A37 A38 A39 A40 A41 A42 A43 A44 A45 A46 A47 A48 A49 A50 A51 A52 A53 A54 A55 A56 A57 A58 A59 A60 A61 A62 A63 A64 A65 A66 A67 A68 A69 A70 A71 A72 A73 A74 A75 A76 A77 A78 A79 A80 A81 A82 A83 A84 A85 A86 A87 A88 A89 A90 A91 A92 A93 A94 A95 A96 A97 A98 A99 A100 A101 A102 A103 A104 A105 A106 L244 L245 L246 L247 L248 L249 L250 L251 L252 L253 | L181 L182 L217 L218 L219 L220 L221 L222 L223 L241 L242 L243 | L181 L182 L212 L213 L214 L215 L216 L236 L237 L238 L239 L240 | L181 L182 L206 L207 L208 L209 L210 L211 L232 L233 L234 L235 | L181 L182 L200 L201 L202 L203 L204 L205 L228 L229 L230 L231 | L181 L182 L194 L195 L196 L197 L198 L199 L224 L225 L226 L227
scale "Scale1" factor 0.2 about (-19.994, -120, 100) bodies 1
